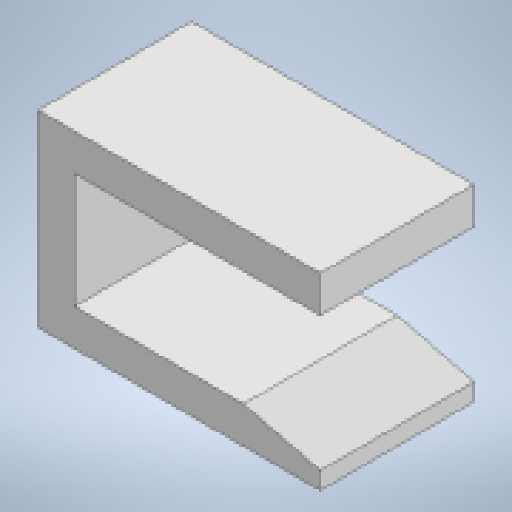
# Autodesk Inventor part: MolexClipper
Saved by Autodesk Inventor 2025.1 (Build 291241000, 241)
## iProperties
Created: 2026-05-09
Part Number: MolexClipper
Material: Generic
Document SubType Name: Modeling
Designer: User
Density: 1 g/cm^3
Appearance: Default
Author: User
Autodesk Inventor part; units mm, degrees
ref_plane "YZ Plane" through (0, 0, 0) normal (1, 0, 0) x (0, 1, 0)
ref_plane "XZ Plane" through (0, 0, 0) normal (0, 1, 0) x (-1, 0, 0)
ref_plane "XY Plane" through (0, 0, 0) normal (0, 0, 1) x (1, 0, 0)
ref_plane "Work Plane1" through (-4.78, -2.9, 8) normal (0, 0, 1) x (1, 0, 0)
sketch "Sketch1" plane through (0, 0, 0) normal (0, 0, 1) x (1, 0, 0)
  line L0 (-6.35, 2.9) -> (-6.35, -2.9)
  line L1 (6.35, 2.9) -> (-6.35, 2.9)
  line L2 (-6.35, -2.9) -> (-5.08, -2.9)
  line L3 (-4.78, -2.9) -> (4.78, -2.9)
  line L4 (-4.78, -2.9) -> (-5.08, -2.9)
  line L5 (5.08, -2.9) -> (6.35, -2.9)
  line L6 (5.08, -2.9) -> (4.78, -2.9)
  line L7 (6.35, 3) -> (-6.45, 3)
  line L8 (-6.45, 3) -> (-6.45, -3)
  line L9 (-6.45, -3) -> (-5.08, -3)
  line L10 (-5.08, -3) -> (-4.78, -3)
  line L11 (-4.78, -3) -> (4.78, -3)
  line L12 (4.78, -3) -> (5.08, -3)
  line L13 (5.08, -3) -> (6.35, -3)
  line L14 (6.35, 4.9) -> (-8.35, 4.9)
  line L15 (-8.35, 4.9) -> (-8.35, -4.9)
  line L16 (-8.35, -4.9) -> (-5.08, -4.9)
  line L17 (-5.08, -4.9) -> (-4.78, -4.9)
  line L18 (-4.78, -4.9) -> (4.78, -4.9)
  line L19 (4.78, -4.9) -> (5.08, -4.9)
  line L20 (5.08, -4.9) -> (6.35, -4.9)
  line L21 (6.35, 4.9) -> (6.35, 3)
  line L22 (6.35, -3) -> (6.35, -4.9)
  point P0 (0, 0)
extrude "Extrusion1" add sketch "Sketch1" along normal up to surface (8 mm away)
chamfer "Chamfer1" distance 1 distance2 4 1 edges at (6.35, -3, 4) measured on face at (6.35, -3.5, 4)
body "Solid1"
